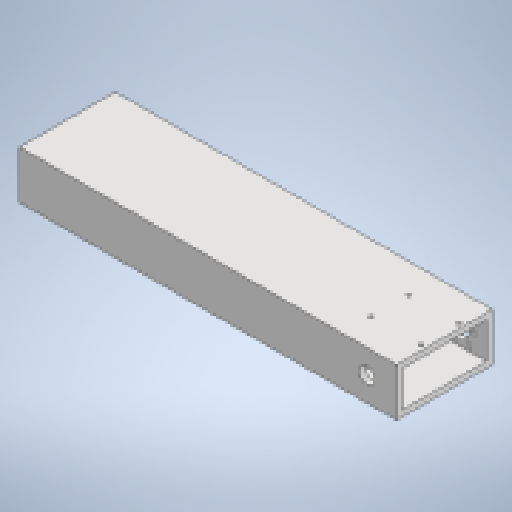
# Autodesk Inventor part: VERTICALTUBE
Saved by Autodesk Inventor 2023 (Build 270158000, 158)
## iProperties
Created: 2022-05-01
Part Number: VERTICALTUBE
Material: Generic
Document SubType Name: Modeling
Designer: plebbb
Density: 1 g/cm^3
Appearance: Default
Author: plebbb
Autodesk Inventor part; units mm, degrees
ref_plane "YZ Plane" through (0, 0, 0) normal (1, 0, 0) x (0, 1, 0)
ref_plane "XZ Plane" through (0, 0, 0) normal (0, 1, 0) x (-1, 0, 0)
ref_plane "XY Plane" through (0, 0, 0) normal (0, 0, 1) x (1, 0, 0)
sketch "Sketch1" plane through (0, 0, 0) normal (1, 0, 0) x (0, 1, 0)
  line L0 (0, 0) -> (50.8, 0)
  line L1 (50.8, 0) -> (50.8, -101.6)
  line L2 (50.8, -101.6) -> (0, -101.6)
  line L3 (0, -101.6) -> (0, 0)
  dimension "d0" = 101.6
  dimension "d1" = 50.8
  constraints: 8 end point, 2 parallel, 1 coincident, 1 horizontal, 1 perpendicular
  measures "d0" distance of L0.end L1.end
  measures "d1" distance of L1.end L2.end
extrude "Extrusion1" add sketch "Sketch1" along normal blind 400
shell "Shell1" thickness 6.35 removed faces 2 at (0, 16.9333, -33.8667) at (400, 16.9333, -33.8667)
sketch "Sketch2" plane through (0, 50.8, 0) normal (0, 1, 0) x (1, 0, 0)
  circle A0 centre (395, 70.8) radius 2
  circle A1 centre (395, 30.8) radius 2
  circle A2 centre (342, 70.8) radius 2
  circle A3 centre (342, 30.8) radius 2
  line L0 (395, 70.8) -> (342, 70.8) construction
  line L1 (342, 70.8) -> (342, 30.8) construction
  line L2 (342, 30.8) -> (395, 30.8) construction
  line L3 (395, 30.8) -> (395, 70.8) construction
  line L4 (400, 101.6) -> (400, 0) projected
  line L5 (337, 101.6) -> (337, 0)
  line L6 (337, 0) -> (400, 0)
  line L7 (400, 101.6) -> (337, 101.6)
  point P0 (368.5, 0)
  point P1 (368.5, 30.8)
  point P2 (395, 50.8)
  point P3 (400, 50.8)
  dimension "d5" = 4
  dimension "d6" = 63
  dimension "d7" = 40
  dimension "d8" = 53
  constraints: 14 end point, 4 centre point, 4 coincident, 4 midpoint, 3 equal radius, 3 horizontal alignment, 2 parallel, 1 horizontal, 1 perpendicular, 1 vertical alignment
  measures "d5" diameter of A1
  measures "d6" distance between parallel lines of L4 L5
  measures "d7" distance of L2.end L0.start
  measures "d8" distance of L1.end L2.end
extrude "Extrusion2" cut sketch "Sketch2" against normal up to surface (6.35 mm away) contours A0 | A1 | A2 | A3
sketch "Sketch3" plane through (0, 0, -101.6) normal (0, 0, 1) x (1, 0, 0)
  line L0 (397, 44.45) -> (393, 44.45) construction
  line L1 (344, 44.45) -> (340, 44.45) construction
  circle A0 centre (368.5, 25.4) radius 19 construction
  line L2 (400, 50.8) -> (400, 0) construction
  line L3 (393, 44.45) -> (368.5, 25.4) construction
  line L4 (368.5, 25.4) -> (344, 44.45) construction
  circle A1 centre (355.065, 11.965) radius 2
  circle A2 centre (381.935, 11.965) radius 2
  circle A3 centre (381.935, 38.835) radius 2
  circle A4 centre (387.5, 25.4) radius 2
  circle A5 centre (355.065, 38.835) radius 2
  circle A6 centre (349.5, 25.4) radius 2
  line L5 (349.5, 25.4) -> (368.5, 25.4) construction
  line L6 (355.065, 11.965) -> (368.5, 25.4) construction
  circle A7 centre (368.5, 25.4) radius 14
  point P0 (0, 0)
  point P1 (400, 25.4)
  point P2 (400, 25.4)
  dimension "d11" = 38
  dimension "d12" = 4
  dimension "d13" = 45
  dimension "d14" = 28
  constraints: 8 centre point, 8 end point, 6 point on circle, 5 equal radius, 4 horizontal alignment, 2 midpoint, 2 vertical alignment, 1 coincident, 1 equal length, 1 horizontal
  measures "d11" diameter of A0
  measures "d12" diameter of A4
  measures "d13" angle of L5 L6
  measures "d14" diameter of A7
extrude "Extrusion3" cut sketch "Sketch3" along normal up to surface (95.25 mm away)
sketch "Sketch4" plane through (0, 0, 0) normal (0, 0, -1) x (-1, 0, 0)
  circle A0 centre (-368.5, 25.4) radius 8.25
  circle A1 centre (-368.5, 25.4) radius 14 projected
  point P0 (0, 0)
  dimension "d17" = 16.5
  constraints: 1 centre point, 1 concentric
  measures "d17" diameter of A0
extrude "Extrusion4" cut sketch "Sketch4" along normal up to surface (95.25 mm away) contours A0
sketch "Sketch5" plane through (0, 0, -101.6) normal (0, -1, 0) x (1, 0, 0)
  circle A0 centre (342, 30.8) radius 2 projected
  circle A1 centre (342, 70.8) radius 2 projected
  circle A2 centre (342, 30.8) radius 5
  circle A3 centre (342, 70.8) radius 5
  point P0 (0, 101.6)
  dimension "d20" = 10
  constraints: 2 centre point, 2 coincident, 1 equal radius
  measures "d20" diameter of A2
extrude "Extrusion5" cut sketch "Sketch5" against normal up to surface (6.35 mm away) contours A0 | A1 | A2 | A3
body "Solid1"
